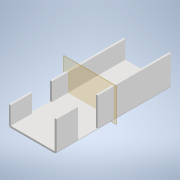
# Autodesk Inventor part: 2020 Front Plate
Saved by Autodesk Inventor 2020.2 (Build 242310000, 310)
## iProperties
Created: 2020-01-12
Part Number: 2020 Front Plate
Material: Generic
Document SubType Name: Modeling
Designer: robst
Density: 1 g/cm^3
Appearance: Default
Author: robst
Autodesk Inventor part; units mm, degrees
ref_plane "YZ Plane" through (0, 0, 0) normal (1, 0, 0) x (0, 1, 0)
ref_plane "XZ Plane" through (0, 0, 0) normal (0, 1, 0) x (-1, 0, 0)
sketch "Sketch1" plane through (0, 0, 0) normal (0, 0, 1) x (1, 0, 0)
  line L0 (0, 3.937) -> (0, 34.925)
  line L1 (0, 34.925) -> (3.175, 34.925)
  line L2 (3.175, 34.925) -> (3.175, 3.175)
  line L3 (3.175, 3.175) -> (81.407, 3.175)
  line L4 (81.407, 3.175) -> (81.407, 53.975)
  line L5 (81.407, 53.975) -> (84.582, 53.975)
  line L6 (84.582, 53.975) -> (84.582, 3.937)
  line L7 (80.645, 0) -> (3.937, 0)
  arc A0 (80.645, 0) -> (84.582, 3.937) centre (80.645, 3.937) ccw
  arc A1 (0, 3.937) -> (3.937, 0) centre (3.937, 3.937) ccw
  point P0 (0, 0)
  dimension "d0" = 34.925
  dimension "d1" = 3.175
  dimension "d2" = 31.75
  dimension "d3" = 78.232
  dimension "d4" = 50.8
  dimension "d5" = 3.175
  dimension "d6" = 3.937
  dimension "d7" = 3.937
  constraints: 16 end point, 7 perpendicular, 4 point on circle, 4 tangent, 2 centre point, 2 point on line, 1 vertical
  measures "d0" distance of point (0, 0) L0.end
  measures "d1" distance of L0.end L1.end
  measures "d2" distance of L1.end L2.end
  measures "d3" distance of L2.end L3.end
  measures "d4" distance of L3.end L4.end
  measures "d5" distance of L4.end L5.end
  measures "d6" radius of A0
  measures "d7" radius of A1
extrude "Extrusion1" add sketch "Sketch1" along normal mid plane 203.2
sketch "Sketch2" plane through (84.582, 3.937, 101.6) normal (1, 0, 0) x (0, 0, -1)
  line L0 (203.2, -0.762) -> (0, -0.762) projected
  line L1 (203.2, 50.038) -> (0, 50.038) projected
  line L2 (73.025, -0.762) -> (38.1, -0.762)
  line L3 (38.1, -0.762) -> (38.1, 50.038)
  line L4 (38.1, 50.038) -> (73.025, 50.038)
  line L5 (73.025, 50.038) -> (73.025, -0.762)
  line L6 (0, 0) -> (0, 50.038) projected
  point P0 (101.6, -3.937)
  point P1 (38.1, -0.762)
  dimension "d10" = 38.1
  dimension "d11" = 34.925
  constraints: 8 end point, 2 parallel, 2 point on line, 1 horizontal, 1 perpendicular
  measures "d10" distance between parallel lines of L3 L6
  measures "d11" distance between parallel lines of L5 L3
extrude "Extrusion2" cut sketch "Sketch2" against normal through all
body "Solid1"
